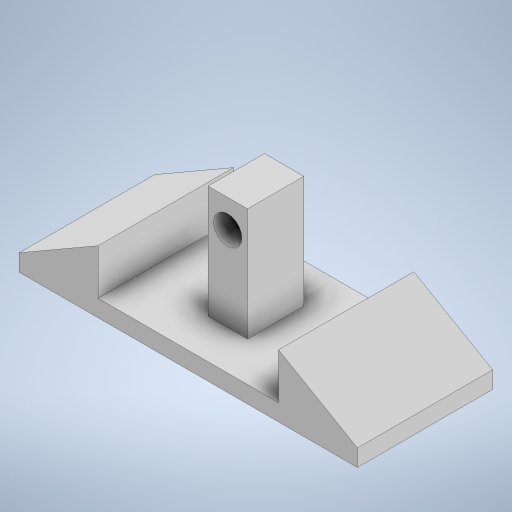
# Autodesk Inventor part: sole_practice
Saved by Autodesk Inventor 2024.3 (Build 283343000, 343)
## iProperties
Created: 2024-10-23
Part Number: sole_practice
Material: 一般
Document SubType Name: Modeling
Designer: 佐藤智貴
Density: 1 g/cm^3
Appearance: 既定
Author: 佐藤智貴
Autodesk Inventor part; units mm, degrees
ref_plane "YZ Plane" through (0, 0, 0) normal (1, 0, 0) x (0, 1, 0)
ref_plane "XZ Plane" through (0, 0, 0) normal (0, 1, 0) x (-1, 0, 0)
ref_plane "XY Plane" through (0, 0, 0) normal (0, 0, 1) x (1, 0, 0)
sketch "スケッチ1" plane through (0, 0, 0) normal (0, 0, 1) x (1, 0, 0)
  line L0 (0, 0) -> (7, 0)
  line L1 (7, 0) -> (7, 20)
  line L2 (7, 20) -> (0, 20)
  line L3 (0, 20) -> (0, 0)
  dimension "d0" = 20
  dimension "d1" = 7
  constraints: 8 end point, 2 parallel, 1 horizontal, 1 perpendicular
  measures "d0" distance of L0.end L1.end
  measures "d1" distance between parallel lines of L3 L1
extrude "押し出し1" add sketch "スケッチ1" along normal blind 10
sketch "スケッチ2" plane through (0, 0, 10) normal (0, 0, 1) x (1, 0, 0)
  circle A0 centre (3.5, 15) radius 2.5
  line L0 (0, 0) -> (7, 0) projected
  line L1 (0, 20) -> (0, 0) projected
  line L2 (7, 20) -> (0, 20) projected
  dimension "d4" = 5
  dimension "d6" = 3.5
  dimension "d15" = 5
  constraints: 1 centre point
  measures "d4" diameter of A0
  measures "d6" distance from line of L1 A0.centre
  measures "d15" distance from line of L2 A0.centre
extrude "押し出し2" cut sketch "スケッチ2" against normal blind 10
sketch "スケッチ3" plane through (0, 0, 0) normal (0, -1, 0) x (1, 0, 0)
  line L0 (33.5, 17) -> (-26.5, 17)
  line L1 (-26.5, 17) -> (-26.5, -7)
  line L2 (-26.5, -7) -> (33.5, -7)
  line L3 (33.5, -7) -> (33.5, 17)
  line L4 (7, 0) -> (0, 0) projected
  line L5 (3.5, 0) -> (3.5, 10)
  line L6 (0, 10) -> (7, 10) projected
  line L7 (7, 0) -> (7, 10) projected
  line L8 (7, 5) -> (0, 5)
  dimension "d9" = 12
  dimension "d10" = 12
  dimension "d11" = 30
  dimension "d12" = 30
  constraints: 12 end point, 3 midpoint, 2 horizontal, 2 parallel, 1 perpendicular
  measures "d9" distance between parallel lines of L0 L8
  measures "d10" distance between parallel lines of L8 L2
  measures "d11" distance between parallel lines of L5 L3
  measures "d12" distance between parallel lines of L1 L5
extrude "押し出し3" add sketch "スケッチ3" along normal blind 3 contours L3 L2 L1 L0 | L4 L5 L8 L7 | L8 L5 L6 L7
sketch "スケッチ4" plane through (-26.5, 0, 17) normal (0, 0, 1) x (1, 0, 0)
  line L0 (60, 0) -> (0, 0) projected
  line L1 (0, 0) -> (14, 8.0829)
  line L2 (14, 8.0829) -> (14, 0)
  line L3 (60, 0) -> (46, 8.0829)
  line L4 (46, 8.0829) -> (46, 0)
  point P0 (26.5, 0)
  dimension "d16" = 60
  dimension "d17" = 60
  dimension "d22" = 14
  dimension "d23" = 14
  constraints: 8 end point, 2 point on line, 1 parallel, 1 vertical
  measures "d16" angle of L2 L1
  measures "d17" angle of L4 L3
  measures "d22" distance from line of L0.start L4
  measures "d23" distance from line of L0.end L2
extrude "押し出し4" add sketch "スケッチ4" against normal blind 24
equation "\"d9\" = d10"
equation "\"d11\" = d12"
equation "\"d17\" = d16"
